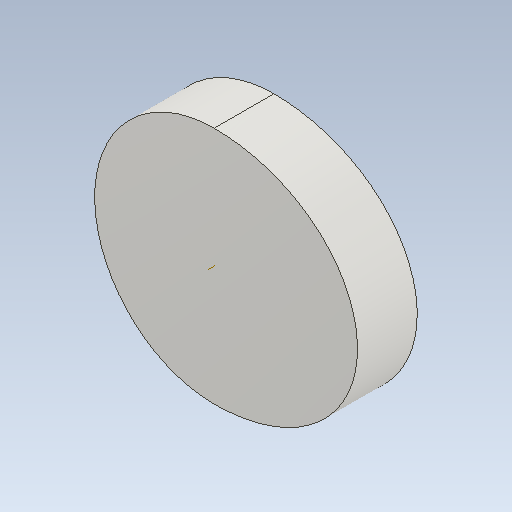
# Autodesk Inventor part: Disc Cam
Saved by Autodesk Inventor 2021.1 (Build 251245000, 245)
## iProperties
Created: 2020-09-02
Part Number: Disc Cam
Material: Stainless Steel, Austenitic
Document SubType Name: Modeling
Designer: robst
Manufacturer: Standard
Standards Organization: Custom
Density: 1 g/cm^3
Appearance: Steel
CustomPartVersion: 1
Author: robst
Autodesk Inventor part; units mm, degrees
ref_plane "YZ Plane" through (0, 0, 0) normal (1, 0, 0) x (0, 1, 0)
ref_plane "XZ Plane" through (0, 0, 0) normal (0, 1, 0) x (-1, 0, 0)
ref_plane "XY Plane" through (0, 0, 0) normal (0, 0, 1) x (1, 0, 0)
sketch "Main Sketch" plane through (0, 0, 0) normal (0, 0, 1) x (1, 0, 0)
  spline S0 degree 5 poles (0, 12.7) (0.3645, 12.701) (0.9957, 12.6849) (2.003, 12.619) (3.2055, 12.4571) (4.772, 12.1195) (6.1873, 11.6796) (7.615, 11.0942) (8.9528, 10.3871) (10.1975, 9.5636) (11.3307, 8.6312) (12.3415, 7.5987) (13.2176, 6.4768) (13.949, 5.2778) (14.5271, 4.0154) (14.9449, 2.7043) (15.1976, 1.3605) (15.2822, 0) (15.1976, -1.3605) (14.9449, -2.7043) (14.5271, -4.0154) (13.949, -5.2778) (13.2176, -6.4768) (12.3415, -7.5987) (11.3307, -8.6312) (10.1975, -9.5636) (8.9529, -10.3871) (7.6147, -11.0942) (6.188, -11.6796) (4.7159, -12.1365) (3.1666, -12.4645) (1.6866, -12.659) (0.0189, -12.7335) (-1.2492, -12.674) (-2.6416, -12.4609) (-3.9249, -12.1137) (-5.1822, -11.6338) (-6.3664, -11.0288) (-7.4858, -10.3027) (-8.5211, -9.4639) (-9.4639, -8.5213) (-10.3027, -7.4854) (-11.0287, -6.3674) (-11.6339, -5.1797) (-12.1116, -3.9353) (-12.4566, -2.6477) (-12.6651, -1.3312) (-12.7349, 0) (-12.6651, 1.3312) (-12.4566, 2.6477) (-12.1116, 3.9353) (-11.6339, 5.1797) (-11.0287, 6.3674) (-10.3027, 7.4854) (-9.464, 8.5213) (-8.521, 9.4639) (-7.486, 10.3027) (-6.366, 11.0288) (-5.183, 11.6337) (-3.9779, 12.0928) (-2.716, 12.4433) (-1.6215, 12.6177) (-0.8687, 12.6824) (-0.3334, 12.699) (0, 12.7) knots 0 0 0 0 0 0 0.021326 0.035498 0.053165 0.07074 0.088202 0.105534 0.12273 0.139787 0.156709 0.173503 0.190185 0.206771 0.223282 0.23974 0.256173 0.272606 0.289064 0.305575 0.322161 0.338843 0.355637 0.372559 0.389616 0.406812 0.424144 0.441606 0.459181 0.476848 0.494271 0.511425 0.528292 0.544856 0.561111 0.577367 0.593622 0.609877 0.626132 0.642387 0.658642 0.674897 0.691152 0.707408 0.723663 0.739918 0.756173 0.772428 0.788683 0.804938 0.821194 0.837449 0.853704 0.869959 0.886214 0.902469 0.918724 0.934979 0.951235 0.96749 0.980494 1 1 1 1 1 1
  point P0 (3.1682, 12.4332)
  point P1 (4.7081, 12.1014)
  point P2 (6.1961, 11.6402)
  point P3 (7.616, 11.0529)
  point P4 (8.9526, 10.3442)
  point P5 (10.1915, 9.5203)
  point P6 (11.3194, 8.5885)
  point P7 (12.3239, 7.5581)
  point P8 (13.1937, 6.4398)
  point P9 (13.9192, 5.2459)
  point P10 (14.4922, 3.99)
  point P11 (14.9061, 2.6867)
  point P12 (15.1563, 1.3514)
  point P13 (15.24, 0)
  point P14 (15.1563, -1.3514)
  point P15 (14.9061, -2.6867)
  point P16 (14.4922, -3.99)
  point P17 (13.9192, -5.2459)
  point P18 (13.1937, -6.4398)
  point P19 (12.3239, -7.5581)
  point P20 (11.3194, -8.5885)
  point P21 (10.1915, -9.5203)
  point P22 (8.9526, -10.3442)
  point P23 (7.616, -11.0529)
  point P24 (6.1961, -11.6402)
  point P25 (4.7081, -12.1014)
  point P26 (3.1682, -12.4332)
  point P27 (1.593, -12.6332)
  point P28 (0, -12.7)
  point P29 (-1.3275, -12.6304)
  point P30 (-2.6405, -12.4225)
  point P31 (-3.9245, -12.0784)
  point P32 (-5.1656, -11.602)
  point P33 (-6.35, -10.9985)
  point P34 (-7.4649, -10.2745)
  point P35 (-8.498, -9.4379)
  point P36 (-9.4379, -8.498)
  point P37 (-10.2745, -7.4649)
  point P38 (-10.9985, -6.35)
  point P39 (-11.602, -5.1656)
  point P40 (-12.0784, -3.9245)
  point P41 (-12.4225, -2.6405)
  point P42 (-12.6304, -1.3275)
  point P43 (-12.7, 0)
  point P44 (-12.6304, 1.3275)
  point P45 (-12.4225, 2.6405)
  point P46 (-12.0784, 3.9245)
  point P47 (-11.602, 5.1656)
  point P48 (-10.9985, 6.35)
  point P49 (-10.2745, 7.4649)
  point P50 (-9.4379, 8.498)
  point P51 (-8.498, 9.4379)
  point P52 (-7.4649, 10.2745)
  point P53 (-6.35, 10.9985)
  point P54 (-5.1656, 11.602)
  point P55 (-3.9245, 12.0784)
  point P56 (-2.6405, 12.4225)
  point P57 (-1.3275, 12.6304)
  constraints: 60 other
extrude "Cam" add sketch "Main Sketch" along normal blind 6.35
body "Solid1"
